Autodesk Fusion 360 part; units mm, degrees
(part 2 of 2)
sketch "Sketch26" plane through (36.1042, -53.0417, 0) normal (0.562692, -0.826667, 0) x (0.826667, 0.562692, 0)
  line L0 (113.4331, 54.4146) -> (209.1515, 86.3566)
  arc A0 (217.028, 80.1422) -> (209.1515, 86.3566) centre (211.0508, 80.6651) ccw
  line L1 (217.028, 80.1422) -> (212.2648, 25.699)
  line L2 (206.3014, 20.222) -> (115.3461, 20.0138)
  arc A1 (109.3324, 26.0138) -> (115.3461, 20.0138) centre (115.3324, 26.0138) ccw
  line L3 (109.3324, 26.0138) -> (109.3324, 48.7231)
  line L4 (76.1102, 33.6322) -> (76.1102, 26)
  arc A2 (70.1102, 20) -> (76.1102, 26) centre (70.1102, 26) ccw
  line L5 (70.1102, 20) -> (47.2394, 20)
  arc A3 (45.3401, 31.6915) -> (47.2394, 20) centre (47.2394, 26) ccw
  line L6 (45.3401, 31.6915) -> (68.2109, 39.3236)
  arc A4 (76.1102, 33.6322) -> (68.2109, 39.3236) centre (70.1102, 33.6322) ccw
  line L7 (325.0034, 50.001) -> (325.0034, 71.001)
  line L8 (325.0034, 71.001) -> (342.0166, 71.001)
  line L9 (342.0166, 71.001) -> (342.0166, 50.001)
  line L10 (342.0166, 50.001) -> (325.0034, 50.001)
  line L11 (86.1102, 0) -> (86.1102, 20)
  line L12 (86.1102, 20) -> (99.3324, 20)
  line L13 (99.3324, 20) -> (99.3324, 0)
  line L14 (99.3324, 0) -> (345.9536, 0)
  arc A5 (345.9536, 0) -> (349.9536, 4) centre (345.9536, 4) ccw
  line L15 (349.9536, 4) -> (349.9536, 179.6934)
  arc A6 (349.9536, 179.6934) -> (343.8124, 183.0721) centre (345.9536, 179.6934) ccw
  line L16 (343.8124, 183.0721) -> (330.2074, 174.4501)
  arc A7 (330.2074, 174.4501) -> (327.9029, 170.6626) centre (332.8838, 170.2268) ccw
  line L17 (327.9029, 170.6626) -> (314.7216, 20)
  line L18 (314.7216, 20) -> (281.7216, 20)
  line L19 (281.7216, 20) -> (292.1427, 139.1136)
  arc A8 (292.1427, 139.1136) -> (286.0167, 142.8409) centre (288.1579, 139.4622) ccw
  line L20 (286.0167, 142.8409) -> (270.8038, 133.1999)
  arc A9 (270.8038, 133.1999) -> (268.9602, 130.1699) centre (272.945, 129.8213) ccw
  line L21 (268.9602, 130.1699) -> (259.3216, 20)
  line L22 (259.3216, 20) -> (226.3216, 20)
  line L23 (226.3216, 20) -> (233.6643, 103.9275)
  arc A10 (233.6643, 103.9275) -> (228.4133, 108.0704) centre (229.6795, 104.2761) ccw
  line L24 (228.4133, 108.0704) -> (-32.9973, 20.8358)
  line L25 (-32.9973, 20.8358) -> (-36.1703, 30.319)
  arc A11 (-36.1703, 30.319) -> (-41.2328, 32.8431) centre (-39.9636, 29.0498) ccw
  line L26 (-41.2328, 32.8431) -> (-48.2106, 30.5083)
  arc A12 (-48.2106, 30.5083) -> (-50.8865, 26.0548) centre (-46.9414, 26.715) ccw
  line L27 (-50.8865, 26.0548) -> (-47.0854, 3.3398)
  arc A13 (-47.0854, 3.3398) -> (-43.1402, 0) centre (-43.1402, 4) ccw
  line L28 (-43.1402, 0) -> (86.1102, 0)
  arc A14 (113.4331, 54.4146) -> (109.3324, 48.7231) centre (115.3324, 48.7231) ccw
  arc A15 (206.3014, 20.222) -> (212.2648, 25.699) centre (206.2877, 26.222) ccw
sketch "Sketch14" plane through (0, -4.5, 0) normal (0, -1, 0) x (1, 0, 0) in component "MainPanelRight"
  line L0 (164.6795, 54.4146) -> (260.398, 86.3566)
  arc A0 (268.2744, 80.1422) -> (260.398, 86.3566) centre (262.2973, 80.6651) ccw
  line L1 (268.2744, 80.1422) -> (263.5113, 25.699)
  line L2 (257.5478, 20.222) -> (166.5925, 20.0138)
  arc A1 (160.5788, 26.0138) -> (166.5925, 20.0138) centre (166.5788, 26.0138) ccw
  line L3 (160.5788, 26.0138) -> (160.5788, 48.7231)
  line L4 (127.3566, 33.6322) -> (127.3566, 26)
  arc A2 (121.3566, 20) -> (127.3566, 26) centre (121.3566, 26) ccw
  line L5 (121.3566, 20) -> (98.4858, 20)
  arc A3 (96.5865, 31.6915) -> (98.4858, 20) centre (98.4858, 26) ccw
  line L6 (96.5865, 31.6915) -> (119.4574, 39.3236)
  arc A4 (127.3566, 33.6322) -> (119.4574, 39.3236) centre (121.3566, 33.6322) ccw
  line L7 (376.2499, 50.001) -> (376.2499, 71.001)
  line L8 (376.2499, 71.001) -> (393.263, 71.001)
  line L9 (393.263, 71.001) -> (393.263, 50.001)
  line L10 (393.263, 50.001) -> (376.2499, 50.001)
  line L11 (137.3566, 0) -> (137.3566, 20)
  line L12 (137.3566, 20) -> (150.5788, 20)
  line L13 (150.5788, 20) -> (150.5788, 0)
  line L14 (150.5788, 0) -> (397.2, 0)
  arc A5 (397.2, 0) -> (401.2, 4) centre (397.2, 4) ccw
  line L15 (401.2, 4) -> (401.2, 179.6934)
  arc A6 (401.2, 179.6934) -> (395.0588, 183.0721) centre (397.2, 179.6934) ccw
  line L16 (395.0588, 183.0721) -> (381.4538, 174.4501)
  arc A7 (381.4538, 174.4501) -> (379.1493, 170.6626) centre (384.1303, 170.2268) ccw
  line L17 (379.1493, 170.6626) -> (365.9681, 20)
  line L18 (365.9681, 20) -> (332.9681, 20)
  line L19 (332.9681, 20) -> (343.3891, 139.1136)
  arc A8 (343.3891, 139.1136) -> (337.2632, 142.8409) centre (339.4044, 139.4622) ccw
  line L20 (337.2632, 142.8409) -> (322.0503, 133.1999)
  arc A9 (322.0503, 133.1999) -> (320.2067, 130.1699) centre (324.1914, 129.8213) ccw
  line L21 (320.2067, 130.1699) -> (310.5681, 20)
  line L22 (310.5681, 20) -> (277.5681, 20)
  line L23 (277.5681, 20) -> (284.9108, 103.9275)
  arc A10 (284.9108, 103.9275) -> (279.6598, 108.0704) centre (280.926, 104.2761) ccw
  line L24 (279.6598, 108.0704) -> (18.2492, 20.8358)
  line L25 (18.2492, 20.8358) -> (15.0761, 30.319)
  arc A11 (15.0761, 30.319) -> (10.0136, 32.8431) centre (11.2828, 29.0498) ccw
  line L26 (10.0136, 32.8431) -> (3.0358, 30.5083)
  arc A12 (3.0358, 30.5083) -> (0.3599, 26.0548) centre (4.305, 26.715) ccw
  line L27 (0.3599, 26.0548) -> (4.1611, 3.3398)
  arc A13 (4.1611, 3.3398) -> (8.1062, 0) centre (8.1062, 4) ccw
  line L28 (8.1062, 0) -> (137.3566, 0)
  line L29 (236.4375, 14.5) -> (248.3789, 14.5)
  line L30 (248.3789, 14.5) -> (248.3789, 5.5)
  line L31 (248.3789, 5.5) -> (236.4375, 5.5)
  line L32 (236.4375, 5.5) -> (236.4375, 14.5)
  arc A14 (164.6795, 54.4146) -> (160.5788, 48.7231) centre (166.5788, 48.7231) ccw
  arc A15 (257.5478, 20.222) -> (263.5113, 25.699) centre (257.5341, 26.222) ccw
  point P0 (236.4375, 14.5)
  point P1 (248.3789, 14.5)
  point P2 (248.3789, 5.5)
  point P3 (236.4375, 5.5)
  constraint horizontal L29
  constraint vertical L30
  constraint horizontal L31
  constraint vertical L32
  constraint coincident P2 L30.end
  constraint coincident P0 L29.start
extrude "Extrude30" cut sketch "Sketch14" against normal blind 9 contours L29 L30 L31 L32 bodies 1 in component "MainPanelRight"
sketch "Sketch27" plane through (38.7573, 56.9394, 0) normal (0.562692, 0.826667, 0) x (-0.826667, 0.562692, 0)
  line L0 (-205.9421, 86.3566) -> (-110.2237, 54.4146)
  arc A0 (-106.123, 48.7231) -> (-110.2237, 54.4146) centre (-112.123, 48.7231) ccw
  line L1 (-106.123, 48.7231) -> (-106.123, 26)
  arc A1 (-112.123, 20) -> (-106.123, 26) centre (-112.123, 26) ccw
  line L2 (-112.123, 20) -> (-203.0588, 20)
  arc A2 (-209.036, 25.4771) -> (-203.0588, 20) centre (-203.0588, 26) ccw
  line L3 (-209.036, 25.4771) -> (-213.8186, 80.1422)
  arc A3 (-205.9421, 86.3566) -> (-213.8186, 80.1422) centre (-207.8414, 80.6651) ccw
  line L4 (-338.8072, 70.9478) -> (-321.794, 70.9478)
  line L5 (-321.794, 70.9478) -> (-321.794, 49.9478)
  line L6 (-321.794, 49.9478) -> (-338.8072, 49.9478)
  line L7 (-338.8072, 49.9478) -> (-338.8072, 70.9478)
  line L8 (-82.9008, 60.5828) -> (-82.9008, 20)
  line L9 (-82.9008, 20) -> (-96.123, 20)
  line L10 (-96.123, 20) -> (-96.123, 64.9951)
  line L11 (-96.123, 64.9951) -> (-225.2039, 108.0704)
  arc A4 (-225.2039, 108.0704) -> (-230.4549, 103.9275) centre (-226.4701, 104.2761) ccw
  line L12 (-230.4549, 103.9275) -> (-223.1122, 20)
  line L13 (-223.1122, 20) -> (-256.1122, 20)
  line L14 (-256.1122, 20) -> (-265.7509, 130.1711)
  arc A5 (-265.7509, 130.1711) -> (-267.5945, 133.2011) centre (-269.7357, 129.8225) ccw
  line L15 (-267.5945, 133.2011) -> (-282.8074, 142.8425)
  arc A6 (-282.8074, 142.8425) -> (-288.9334, 139.1153) centre (-284.9487, 139.4639) ccw
  line L16 (-288.9334, 139.1153) -> (-278.5122, 20)
  line L17 (-278.5122, 20) -> (-311.5122, 20)
  line L18 (-311.5122, 20) -> (-324.6921, 170.6469)
  arc A7 (-324.6921, 170.6469) -> (-326.9965, 174.4344) centre (-329.6731, 170.2111) ccw
  line L19 (-326.9965, 174.4344) -> (-340.6029, 183.0577)
  arc A8 (-340.6029, 183.0577) -> (-346.7442, 179.6791) centre (-342.7442, 179.6791) ccw
  line L20 (-346.7442, 179.6791) -> (-346.7442, 4)
  arc A9 (-346.7442, 4) -> (-342.7442, 0) centre (-342.7442, 4) ccw
  line L21 (-342.7442, 0) -> (46.3496, 0)
  arc A10 (46.3496, 0) -> (50.2948, 3.3398) centre (46.3496, 4) ccw
  line L22 (50.2948, 3.3398) -> (54.0959, 26.0548)
  arc A11 (54.0959, 26.0548) -> (51.42, 30.5083) centre (50.1508, 26.715) ccw
  line L23 (51.42, 30.5083) -> (44.4422, 32.8431)
  arc A12 (44.4422, 32.8431) -> (39.3797, 30.319) centre (43.173, 29.0498) ccw
  line L24 (39.3797, 30.319) -> (36.2067, 20.8358)
  line L25 (36.2067, 20.8358) -> (-82.9008, 60.5828)
  line L26 (-193.9231, 14.5) -> (-181.9817, 14.5)
  line L27 (-181.9817, 14.5) -> (-181.9817, 5.5)
  line L28 (-181.9817, 5.5) -> (-193.9231, 5.5)
  line L29 (-193.9231, 5.5) -> (-193.9231, 14.5)
  line L30 (-44.03, 20) -> (-66.9008, 20)
  arc A13 (-72.9008, 26) -> (-66.9008, 20) centre (-66.9008, 26) ccw
  line L31 (-72.9008, 26) -> (-72.9008, 33.6322)
  arc A14 (-65.0015, 39.3236) -> (-72.9008, 33.6322) centre (-66.9008, 33.6322) ccw
  line L32 (-65.0015, 39.3236) -> (-42.1307, 31.6915)
  arc A15 (-44.03, 20) -> (-42.1307, 31.6915) centre (-44.03, 26) ccw
  point P0 (-193.9231, 14.5)
  point P1 (-181.9817, 5.5)
  constraint horizontal L26
  constraint vertical L27
  constraint horizontal L28
  constraint vertical L29
  constraint coincident P1 L27.end
  constraint coincident P0 L26.start
extrude "Extrude30'" cut sketch "Sketch27" against normal blind 9 contours L26 L27 L28 L29 sketch seen with x (0.826667, 0.562692, 0) y (-0.562692, 0.826667, 0) z (0, 0, 1) at (54.4558, -64.3784, 0) bodies 2 in component "MainPanelLeft"
sketch "rounded-middle-bar" plane through (33.6931, 49.4994, 0) normal (-0.562692, -0.826667, 0) x (0.826667, -0.562692, 0)
  line L0 (181.9817, 5.5) -> (181.9817, 14.5)
  line L1 (181.9817, 14.5) -> (193.9231, 14.5)
  line L2 (193.9231, 14.5) -> (193.9231, 5.5)
  line L3 (193.9231, 5.5) -> (181.9817, 5.5)
  line L4 (110.2237, 54.4146) -> (205.9421, 86.3566)
  arc A0 (213.8186, 80.1422) -> (205.9421, 86.3566) centre (207.8414, 80.6651) ccw
  line L5 (213.8186, 80.1422) -> (209.036, 25.4771)
  arc A1 (203.0588, 20) -> (209.036, 25.4771) centre (203.0588, 26) ccw
  line L6 (203.0588, 20) -> (112.123, 20)
  arc A2 (106.123, 26) -> (112.123, 20) centre (112.123, 26) ccw
  line L7 (106.123, 26) -> (106.123, 48.7231)
  arc A3 (110.2237, 54.4146) -> (106.123, 48.7231) centre (112.123, 48.7231) ccw
  line L8 (66.9008, 20) -> (44.03, 20)
  arc A4 (42.1307, 31.6915) -> (44.03, 20) centre (44.03, 26) ccw
  line L9 (42.1307, 31.6915) -> (65.0015, 39.3236)
  arc A5 (72.9008, 33.6322) -> (65.0015, 39.3236) centre (66.9008, 33.6322) ccw
  line L10 (72.9008, 33.6322) -> (72.9008, 26)
  arc A6 (66.9008, 20) -> (72.9008, 26) centre (66.9008, 26) ccw
  line L11 (321.794, 70.9478) -> (338.8072, 70.9478)
  line L12 (338.8072, 70.9478) -> (338.8072, 49.9478)
  line L13 (338.8072, 49.9478) -> (321.794, 49.9478)
  line L14 (321.794, 49.9478) -> (321.794, 70.9478)
  line L15 (82.9008, 20) -> (82.9008, 60.5828)
  line L16 (82.9008, 60.5828) -> (-36.2067, 20.8358)
  line L17 (-36.2067, 20.8358) -> (-39.3797, 30.319)
  arc A7 (-39.3797, 30.319) -> (-44.4422, 32.8431) centre (-43.173, 29.0498) ccw
  line L18 (-44.4422, 32.8431) -> (-51.42, 30.5083)
  arc A8 (-51.42, 30.5083) -> (-54.0959, 26.0548) centre (-50.1508, 26.715) ccw
  line L19 (-54.0959, 26.0548) -> (-50.2947, 3.3398)
  arc A9 (-50.2947, 3.3398) -> (-46.3496, 0) centre (-46.3496, 4) ccw
  line L20 (-46.3496, 0) -> (342.7442, 0)
  arc A10 (342.7442, 0) -> (346.7442, 4) centre (342.7442, 4) ccw
  line L21 (346.7442, 4) -> (346.7442, 179.6791)
  arc A11 (346.7442, 179.6791) -> (340.6029, 183.0577) centre (342.7442, 179.6791) ccw
  line L22 (340.6029, 183.0577) -> (326.9965, 174.4344)
  arc A12 (326.9965, 174.4344) -> (324.6921, 170.6469) centre (329.6731, 170.2111) ccw
  line L23 (324.6921, 170.6469) -> (311.5122, 20)
  line L24 (311.5122, 20) -> (278.5122, 20)
  line L25 (278.5122, 20) -> (288.9334, 139.1153)
  arc A13 (288.9334, 139.1153) -> (282.8074, 142.8425) centre (284.9487, 139.4639) ccw
  line L26 (282.8074, 142.8425) -> (267.5945, 133.2011)
  arc A14 (267.5945, 133.2011) -> (265.7509, 130.1711) centre (269.7357, 129.8225) ccw
  line L27 (265.7509, 130.1711) -> (256.1122, 20)
  line L28 (256.1122, 20) -> (223.1122, 20)
  line L29 (223.1122, 20) -> (230.4549, 103.9275)
  arc A15 (230.4549, 103.9275) -> (225.2039, 108.0704) centre (226.4701, 104.2761) ccw
  line L30 (225.2039, 108.0704) -> (96.123, 64.9951)
  line L31 (96.123, 64.9951) -> (96.123, 20)
  line L32 (96.123, 20) -> (82.9008, 20)
  line L33 (193.9231, 14.5) -> (181.9817, 14.5)
  line L34 (181.9817, 14.5) -> (181.9817, 5.5)
  line L35 (181.9817, 5.5) -> (193.9231, 5.5)
  line L36 (193.9231, 5.5) -> (193.9231, 14.5)
  line L37 (184.9817, 14.5) -> (190.9231, 14.5)
  line L38 (193.9231, 11.5) -> (193.9231, 8.5)
  line L39 (190.9231, 5.5) -> (184.9817, 5.5)
  line L40 (181.9817, 8.5) -> (181.9817, 11.5)
  arc A16 (184.9817, 14.5) -> (181.9817, 11.5) centre (184.9817, 11.5) ccw
  arc A17 (193.9231, 11.5) -> (190.9231, 14.5) centre (190.9231, 11.5) ccw
  arc A18 (190.9231, 5.5) -> (193.9231, 8.5) centre (190.9231, 8.5) ccw
  arc A19 (181.9817, 8.5) -> (184.9817, 5.5) centre (184.9817, 8.5) ccw
  dimension "d226" = 3
  dimension "d227" = 3
  dimension "d228" = 3
  dimension "d229" = 3
  constraint horizontal L37
  constraint vertical L38
  constraint horizontal L39
  constraint vertical L40
  constraint tangent L37 A16
  constraint tangent L40 A16
  constraint tangent L37 A17
  constraint tangent L38 A17
  constraint tangent L38 A18
  constraint tangent L39 A18
  constraint tangent L40 A19
  constraint tangent L39 A19
  measures "d226" radius of A16
  measures "d227" radius of A17
  measures "d228" radius of A18
  measures "d229" radius of A19
component "MainPanelRight" placed x (0.826667, 0.562692, 0) y (-0.562692, 0.826667, 0) z (0, 0, 1) at (-8.7916, -78.1577, 0)
component "MainPanelLeft" placed x (0.826667, -0.562692, 0) y (0.562692, 0.826667, 0) z (0, 0, 1) at (-8.7916, 83.8613, 0)
hidden bodies 4
equation "b = 260 mm"
equation "angle = acos(310 / 375)"
equation "d3 = b"
equation "thick = 9 mm"
equation "edgerad = 4 mm"
equation "d1 = length + ( 2 * ( 33 - 22.4 ) ) * 1 mm"
equation "length = 380 mm"
equation "width = 260 mm"
equation "thick_1 = 9 mm"
equation "edgerad_1 = 4 mm"
equation "d9_1 = 90 deg - 18.5 deg"
equation "d41 = 180 deg - 18.5 deg"
equation "d66 = 143 mm - thick_1 / 2"
equation "d68 = thick_1"
equation "d129 = edgerad_1"
equation "d131 = edgerad_1"
equation "d134 = edgerad_1"
equation "d137 = edgerad_1"
equation "d138 = edgerad_1"
equation "d139 = edgerad_1"
equation "d142 = edgerad_1"
equation "d143 = edgerad_1"
equation "d147 = thick_1 / 2"
equation "d149 = edgerad_1"
equation "d1_1 = length_1 + ( ( 33 - 22.4 ) * 2 ) * 1 mm"
equation "length_1 = 380 mm"
equation "width_1 = 260 mm"
equation "thick_2 = 9 mm"
equation "edgerad_2 = 4 mm"
equation "d9_2 = 90 deg - 18.5 deg"
equation "d41_1 = 180 deg - 18.5 deg"
equation "d66_1 = 143 mm - thick_2 / 2"
equation "d68_1 = thick_2"
equation "d129_1 = edgerad_2"
equation "d131_1 = edgerad_2"
equation "d134_1 = edgerad_2"
equation "d137_1 = edgerad_2"
equation "d138_1 = edgerad_2"
equation "d139_1 = edgerad_2"
equation "d142_1 = edgerad_2"
equation "d143_1 = edgerad_2"
equation "d147_1 = thick_2 / 2"
equation "d149_1 = edgerad_2"
equation "d43 = thick"
equation "d63 = thick"
equation "d71 = thick"
equation "d75 = -thick"
equation "d87 = -thick"
equation "d102 = -thick"
equation "d110 = -thick"
equation "d167 = -thick"
equation "d169 = -thick"
equation "cableHolderW = 30 mm"
equation "cableHolderBackMove = 8 mm"
equation "cableHolderDia = 6 mm"
equation "d193 = cableHolderW / 2 - cableHolderBackMove"
equation "d197 = cableHolderW"
equation "d198 = cableHolderBackMove"
equation "d200 = cableHolderBackMove"
equation "d202 = cableHolderW"
equation "d203 = cableHolderBackMove"
equation "d205 = cableHolderW"
equation "d206 = cableHolderBackMove"
equation "d208 = cableHolderW"
equation "d209 = cableHolderDia"
equation "d210 = cableHolderDia"
equation "d211 = cableHolderDia"
equation "d212 = cableHolderDia"
equation "d213 = cableHolderDia"
equation "d214 = cableHolderDia"
equation "d215 = cableHolderDia"
equation "d216 = cableHolderDia"
equation "d217 = cableHolderDia"
equation "d218 = cableHolderDia"
equation "d219 = cableHolderDia"
named bodies: "MiddleBar", "BackBarConstructionBody", "BackBar"
